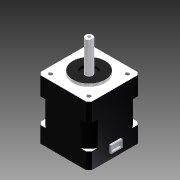
# Autodesk Inventor part: NEMA14 Stepper Motor
Saved by Autodesk Inventor 2012 (Build 160160000, 160)
## iProperties
Created: 2012-06-25
Part Number: NEMA14 Stepper Motor
Material: Default
Document SubType Name: Modeling
Designer: MCP
Density: 1 g/cm^3
Author: MCP
Autodesk Inventor part; units mm, degrees
ref_plane "YZ Plane" through (0, 0, 0) normal (1, 0, 0) x (0, 1, 0)
ref_plane "XZ Plane" through (0, 0, 0) normal (0, 1, 0) x (-1, 0, 0)
ref_plane "XY Plane" through (0, 0, 0) normal (0, 0, 1) x (1, 0, 0)
sketch "Sketch1" plane through (0, 0, 0) normal (0, 1, 0) x (-1, 0, 0)
  line L0 (0, 0) -> (35.052, 0)
  line L1 (35.052, 0) -> (35.052, 35.052)
  line L2 (35.052, 35.052) -> (0, 35.052)
  line L3 (0, 35.052) -> (0, 0)
  dimension "d0" = 35.052
  dimension "d1" = 35.052
  constraints: 8 end point, 2 parallel, 1 horizontal, 1 perpendicular
  measures "d0" distance of L2.end L1.end
  measures "d1" distance of L1.end L0.end
extrude "Extrusion1" add sketch "Sketch1" along normal blind 11.0236
sketch "Sketch2" plane through (0, 11.0236, 0) normal (0, 1, 0) x (1, 0, 0)
  circle A0 centre (-17.526, -17.526) radius 21.0185 construction
  arc A1 (-35.052, -29.1284) -> (-29.1284, -35.052) centre (-17.526, -17.526) ccw
  arc A2 (-5.9236, -35.052) -> (0, -29.1284) centre (-17.526, -17.526) ccw
  arc A3 (0, -5.9236) -> (-5.9236, 0) centre (-17.526, -17.526) ccw
  arc A4 (-29.1284, 0) -> (-35.052, -5.9236) centre (-17.526, -17.526) ccw
  line L0 (-29.1284, 0) -> (-5.9236, 0)
  line L1 (0, -5.9236) -> (0, -29.1284)
  line L2 (-29.1284, -35.052) -> (-5.9236, -35.052)
  line L3 (-35.052, -29.1284) -> (-35.052, -5.9236)
  point P0 (0, -35.052)
  point P1 (-35.052, 0)
  dimension "d4" = 42.037
  constraints: 8 end point, 8 point on circle, 4 centre point, 3 perpendicular, 1 horizontal, 14 other
extrude "Extrusion2" add sketch "Sketch2" along normal blind 16.6878
sketch "Sketch3" plane through (0, 27.7114, 0) normal (0, 1, 0) x (1, 0, 0)
  line L0 (-35.052, 0) -> (0, 0)
  line L1 (0, 0) -> (0, -35.052)
  line L2 (0, -35.052) -> (-35.052, -35.052)
  line L3 (-35.052, -35.052) -> (-35.052, 0)
  constraints: 8 end point, 2 parallel, 1 horizontal, 1 perpendicular
extrude "Extrusion3" add sketch "Sketch3" along normal blind 12.446
chamfer "Chamfer1" distance 2 angle 45 8 edges at (0, 33.9344, 35.052) (-35.052, 5.5118, 35.052) (0, 5.5118, 35.052) (0, 5.5118, 0) (0, 33.9344, 0) (-35.052, 33.9344, 35.052) (-35.052, 33.9344, 0) (-35.052, 5.5118, 0)
sketch "Sketch4" plane through (0, 40.1574, 0) normal (0, 1, 0) x (1, 0, 0)
  circle A0 centre (-17.526, -17.526) radius 10.9728
  circle A1 centre (-17.526, -17.526) radius 5.08
  point P0 (0, 0)
  dimension "d12" = 21.9456
  dimension "d13" = 10.16
  constraints: 2 centre point, 1 coincident
  measures "d12" diameter of A0
  measures "d13" diameter of A1
extrude "Extrusion4" add sketch "Sketch4" along normal blind 1.9558
sketch "Sketch5" plane through (-17.526, 40.1574, 17.526) normal (0, 1, 0) x (1, 0, 0)
  circle A0 centre (0, 0) radius 5.08 projected
  circle A1 centre (0, 0) radius 2.5
  point P0 (17.526, 17.526)
  dimension "d16" = 5
  constraints: 1 centre point, 1 coincident
  measures "d16" diameter of A1
extrude "Extrusion5" add sketch "Sketch5" along normal blind 21.59 contours A1
sketch "Sketch6" plane through (0, 40.1574, 0) normal (0, 1, 0) x (1, 0, 0)
  line L0 (-35.052, -33.052) -> (-35.052, -2) projected
  line L1 (0, -2) -> (0, -33.052) projected
  line L2 (-33.052, 0) -> (-2, 0) projected
  circle A0 centre (-30.5308, -4.5212) radius 1.1938
  circle A1 centre (-4.5308, -4.5212) radius 1.1938
  circle A2 centre (-30.5308, -30.5212) radius 1.1938
  circle A3 centre (-4.5308, -30.5212) radius 1.1938
  point P0 (0, 0)
  dimension "d21" = 2.3876
  dimension "d63" = 26
  dimension "d66" = 26
  dimension "d69" = 4.5212
  dimension "d70" = 4.5308
  dimension "d71" = 4.5212
  constraints: 4 centre point, 1 horizontal, 1 vertical, 6 other
  measures "d21" diameter of A0
  measures "d63" distance of A0.centre A1.centre
  measures "d66" distance of A0.centre A2.centre
  measures "d69" distance from line of L0 A0.centre
  measures "d70" distance from line of L1 A1.centre
  measures "d71" distance from line of L2 A0.centre
extrude "Extrusion6" cut sketch "Sketch6" against normal blind 7.62
chamfer "Chamfer2" distance 0.2 angle 45 41 edges at (-17.526, 0, 35.052) (0, 0, 17.526) (-1, 0, 34.052) (-1, 0, 1) (-17.526, 0, 0) (-34.052, 0, 1) (-35.052, 0, 17.526) (-34.052, 0, 34.052) (-35.052, 11.0236, 31.0902) (-34.052, 11.0236, 34.052) (-31.0902, 11.0236, 35.052) (-3.9618, 11.0236, 35.052) (-1, 11.0236, 34.052) (0, 11.0236, 31.0902) (0, 27.7114, 31.0902) (-1, 27.7114, 34.052) (-3.9618, 27.7114, 35.052) (-31.0902, 27.7114, 35.052) (-34.052, 27.7114, 34.052) (-35.052, 27.7114, 31.0902) (0, 27.7114, 3.9618) (-1, 27.7114, 1) (-3.9618, 27.7114, 0) (-1, 11.0236, 1) (-3.9618, 11.0236, 0) (0, 11.0236, 3.9618) (-17.526, 40.1574, 35.052) (-1, 40.1574, 34.052) (0, 40.1574, 17.526) (-1, 40.1574, 1) (-17.526, 40.1574, 0) (-34.052, 40.1574, 34.052) (-35.052, 40.1574, 17.526) (-34.052, 40.1574, 1) (-31.7246, 40.1574, 4.5212) (-35.052, 11.0236, 3.9618) (-31.0902, 11.0236, 0) (-34.052, 11.0236, 1) (-35.052, 27.7114, 3.9618) (-34.052, 27.7114, 1) (-31.0902, 27.7114, 0)
chamfer "Chamfer3" distance 0.2 angle 45 2 edges at (-20.026, 61.7474, 17.526) (-22.606, 42.1132, 17.526)
sketch "Sketch7" plane through (-17.526, 61.7474, 17.526) normal (0, 1, 0) x (1, 0, 0)
  circle A0 centre (0, 0) radius 2.3 projected
  circle A1 centre (0, 0) radius 1.0795
  point P0 (17.526, 17.526)
  constraints: 1 centre point, 1 coincident
extrude "Extrusion7" cut sketch "Sketch7" against normal blind 2.54 contours A1
thread "Thread4" size "M2.5x0.45" class "6H" standard "ANSI Metric M Profile" full length
sketch "Sketch8" plane through (0, 10.8236, 29.1284) normal (1, 0, 0) x (0, 0, -1)
  line L0 (-3.9236, -10.6236) -> (-3.9236, 0) projected
  line L1 (27.1284, -10.6236) -> (-3.9236, -10.6236) projected
  line L2 (27.1284, 0) -> (27.1284, -10.6236) projected
  line L3 (-3.9236, -6.5596) -> (27.1284, -6.5596) construction
  line L4 (11.6024, -6.5596) -> (15.4378, -6.5596)
  line L5 (11.6024, -6.5596) -> (7.767, -6.5596)
  line L6 (7.767, -6.5596) -> (7.767, -1.4796)
  line L7 (7.767, -1.4796) -> (15.4378, -1.4796)
  line L8 (15.4378, -1.4796) -> (15.4378, -6.5596)
  line L9 (8.656, -2.3686) -> (14.6558, -2.3686)
  line L10 (14.6558, -2.3686) -> (14.6558, -5.7488)
  line L11 (14.6558, -5.7488) -> (8.656, -5.7488)
  line L12 (8.656, -5.7488) -> (8.656, -2.3686)
  point P0 (29.1284, -10.8236)
  dimension "d49" = 4.064
  dimension "d50" = 3.8354
  dimension "d51" = 3.8354
  dimension "d52" = 5.08
  dimension "d53" = 0.889
  dimension "d54" = 0.889
  constraints: 20 end point, 4 perpendicular, 4 point on line, 3 parallel, 1 horizontal, 1 midpoint
  measures "d49" distance between parallel lines of L1 L3
  measures "d50" distance of L4.start L4.end
  measures "d51" distance of L4.start L5.end
  measures "d52" distance of L5.end L6.end
  measures "d53" distance between parallel lines of L7 L9
  measures "d54" distance between parallel lines of L12 L6
extrude "Extrusion8" add sketch "Sketch8" along normal blind 1.27
sketch "Sketch9" plane through (0, 0, 0) normal (0, -1, 0) x (1, 0, 0)
  circle A0 centre (-17.526, 17.526) radius 4.699
  point P0 (0, 0)
  dimension "d57" = 9.398
  constraints: 1 centre point
  measures "d57" diameter of A0
extrude "Extrusion9" cut sketch "Sketch9" against normal blind 1.27
thread "Thread5" size "M3x0.5" class "6H" standard "ANSI Metric M Profile" full length
thread "Thread6" size "M3x0.5" class "6H" standard "ANSI Metric M Profile" full length
thread "Thread7" size "M3x0.5" class "6H" standard "ISO Metric profile" full length
chamfer "Chamfer4" distance 0.254 angle 45 3 edges at (-31.7246, 40.1574, 30.5212) (-5.7246, 40.1574, 30.5212) (-5.7246, 40.1574, 4.5212)
body "Solid1"
